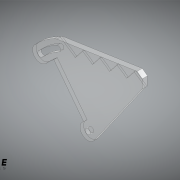
# Autodesk Inventor part: 転倒補助
Saved by Autodesk Inventor 2020 (Build 240168000, 168)
## iProperties
Created: 2019-12-24
Part Number: 転倒補助
Material: ポリカーボネート、クリア
Document SubType Name: Modeling
Designer: tanjihayato
Density: 1.2 g/cm^3
Appearance: ポリカーボネート - クリア
Author: tanjihayato
Autodesk Inventor part; units mm, degrees
ref_plane "YZ Plane" through (0, 0, 0) normal (1, 0, 0) x (0, 1, 0)
ref_plane "XZ Plane" through (0, 0, 0) normal (0, 1, 0) x (-1, 0, 0)
ref_plane "XY Plane" through (0, 0, 0) normal (0, 0, 1) x (1, 0, 0)
sketch "スケッチ1" plane through (0, 0, 0) normal (0, 0, 1) x (1, 0, 0)
  line L0 (174.213, 45.2914) -> (127.5208, 38.2253)
  arc A0 (127.5208, 38.2253) -> (126.1111, 37.7648) centre (128.1942, 33.7759) ccw
  arc A1 (126.1111, 37.7648) -> (114.5668, 28.8826) centre (145.5257, 0.5882) ccw
  arc A2 (114.5668, 28.8826) -> (121.2102, 22.8109) centre (117.8885, 25.8468) ccw
  arc A3 (125.4386, 26.6957) -> (121.2102, 22.8109) centre (145.5257, 0.5882) ccw
  arc A4 (125.4386, 26.6957) -> (125.7514, 26.9599) centre (122.6945, 30.2622) ccw
  line L1 (125.7514, 26.9599) -> (143.1172, 4.3894)
  arc A5 (143.1172, 4.3894) -> (149.2108, -1.9944) centre (145.5257, 0.5882) ccw
  line L2 (149.2108, -1.9944) -> (177.0395, 37.7154)
  line L3 (177.0395, 37.7154) -> (177.2058, 43.0125)
  line L4 (177.2058, 43.0125) -> (174.213, 45.2914)
  circle A6 centre (145.5257, 0.5882) radius 1.5
  arc A7 (116.7813, 26.8587) -> (118.9958, 24.8348) centre (117.8885, 25.8468) ccw
  arc A8 (127.4998, 35.1056) -> (116.7813, 26.8587) centre (145.5257, 0.5882) ccw
  arc A9 (128.8885, 32.4463) -> (127.4998, 35.1056) centre (128.1942, 33.7759) ccw
  arc A10 (128.8885, 32.4463) -> (118.9958, 24.8348) centre (145.5257, 0.5882) ccw
  line L5 (174.213, 45.2914) -> (127.5208, 38.2253)
  line L6 (177.0395, 37.7154) -> (177.2058, 43.0125)
  line L7 (125.7514, 26.9599) -> (143.1172, 4.3894)
  line L8 (127.5208, 38.2253) -> (136.18, 32.2797)
  line L9 (136.18, 32.2797) -> (140.4689, 37.7075)
  line L10 (140.4689, 37.7075) -> (146.1718, 33.7918)
  line L11 (146.1718, 33.7918) -> (150.4607, 39.2196)
  line L12 (150.4607, 39.2196) -> (156.1635, 35.3039)
  line L13 (156.1635, 35.3039) -> (160.4524, 40.7317)
  line L14 (160.4524, 40.7317) -> (166.1553, 36.816)
  line L15 (166.1553, 36.816) -> (170.4442, 42.2438)
  line L16 (136.18, 32.2797) -> (166.1553, 36.816) construction
  line L17 (170.4442, 42.2438) -> (177.0395, 37.7154)
  line L18 (150.0297, -2.5683) -> (177.8584, 37.1415)
  arc A11 (141.7229, 4.5617) -> (150.0297, -2.5683) centre (145.5257, 0.5882) ccw
  line L19 (125.5834, 25.5384) -> (141.7229, 4.5617)
  arc A12 (126.4864, 39.0041) -> (125.6482, 38.6512) centre (128.1942, 33.7759) ccw
  arc A13 (125.6482, 38.6512) -> (113.8286, 29.5572) centre (145.5257, 0.5882) ccw
  arc A14 (113.8286, 29.5572) -> (121.9484, 22.1363) centre (117.8885, 25.8468) ccw
  arc A15 (125.5834, 25.5384) -> (121.9484, 22.1363) centre (145.5257, 0.5882) ccw
  line L20 (177.0395, 37.7154) -> (177.8584, 37.1415)
  line L21 (127.5208, 38.2253) -> (126.4864, 39.0041)
  point P0 (0, 0)
  point P1 (0, 0)
  dimension "d4" = 1
  dimension "d5" = 1
  dimension "d6" = 1
  dimension "d7" = 1
  constraints: 44 end point, 30 point on circle, 16 centre point, 10 parallel, 4 equal length, 2 point on line, 1 other
  measures "d4" distance between parallel lines of L2 L18
  measures "d5" radial gap between concentric circles of A5 A11
  measures "d6" distance between parallel lines of L1 L19
  measures "d7" radial gap between concentric circles of A3 A15
extrude "押し出し1" add sketch "スケッチ1" against normal blind 2 contours L8 L9 L10 L11 L12 L13 L14 L15 L17 L2 A5 L1 A4 A3 A2 A1 A0
extrude "押し出し2" add sketch "スケッチ1" against normal blind 3 contours L4 L3 L17 L15 L14 L13 L12 L11 L10 L9 L8 L0
